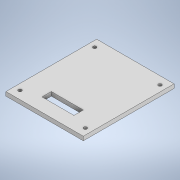
# Autodesk Inventor part: Podkladka
Saved by Autodesk Inventor 2021 (Build 250183000, 183)
## iProperties
Created: 2021-01-18
Part Number: Podkladka
Material: Generic
Document SubType Name: Modeling
Designer: emili
Density: 1 g/cm^3
Appearance: Default
Author: emili
Autodesk Inventor part; units mm, degrees
ref_plane "YZ Plane" through (0, 0, 0) normal (1, 0, 0) x (0, 1, 0)
ref_plane "XZ Plane" through (0, 0, 0) normal (0, 1, 0) x (-1, 0, 0)
ref_plane "XY Plane" through (0, 0, 0) normal (0, 0, 1) x (1, 0, 0)
sketch "Sketch2" plane through (0, 0, 0) normal (0, 1, 0) x (-1, 0, 0)
  line L0 (8, 0) -> (8, -5)
  line L1 (32, 0) -> (32, -5)
  line L2 (32, -5) -> (8, -5)
  line L3 (8, -5) -> (8, 0)
  line L4 (32, 0) -> (32, -5)
  line L5 (-9, 0) -> (-9, 9)
  line L6 (-9, 9) -> (0, 9)
  line L7 (49, -44) -> (49, -53)
  line L8 (49, -53) -> (40, -53)
  line L9 (-9, 9) -> (49, 9)
  line L10 (49, 9) -> (49, -53)
  line L11 (49, -53) -> (-9, -53)
  line L12 (-9, -53) -> (-9, 9)
  line L13 (8, 0) -> (8, 2)
  line L14 (8, 2) -> (32, 2)
  line L15 (32, 2) -> (32, 0)
  line L16 (32, 2) -> (8, 2)
  line L17 (8, 2) -> (8, -5)
  line L18 (8, -5) -> (32, -5)
  line L19 (32, -5) -> (32, 2)
  point P0 (0, 0)
  constraints: 40 end point, 6 parallel, 3 horizontal, 3 perpendicular
extrude "Extrusion1" add sketch "Sketch2" along normal blind 3
sketch "Sketch3" plane through (-49, 0, 9) normal (0, 0, 1) x (1, 0, 0)
  line L0 (0, 0) -> (0, 3) projected
  line L1 (58, 0) -> (58, 3) projected
  line L2 (0, 3) -> (58, 3)
  line L3 (58, 3) -> (58, 0)
  line L4 (58, 0) -> (0, 0)
  line L5 (0, 0) -> (0, 3)
  point P0 (49, 0)
  constraints: 8 end point, 2 parallel, 1 horizontal, 1 perpendicular
extrude "Extrusion2" add sketch "Sketch3" along normal blind 3
sketch "Sketch4" plane through (9, 0, -53) normal (0, 0, -1) x (-1, 0, 0)
  line L0 (58, 3) -> (58, 0) projected
  line L1 (58, 0) -> (0, 0) projected
  line L2 (58, 3) -> (0, 3)
  line L3 (0, 3) -> (0, 0)
  line L4 (0, 0) -> (58, 0)
  line L5 (58, 0) -> (58, 3)
  point P0 (9, 0)
  constraints: 8 end point, 2 parallel, 1 horizontal, 1 perpendicular
extrude "Extrusion3" add sketch "Sketch4" along normal blind 3
sketch "Sketch5" plane through (0, 3, 0) normal (0, 1, 0) x (1, 0, 0)
  line L0 (9, -12) -> (0, -12)
  line L1 (0, -12) -> (0, 0)
  line L2 (0, 0) -> (9, 0)
  line L3 (9, 0) -> (9, -12)
  line L4 (-49, -12) -> (-49, 56) projected
  line L5 (-49, 56) -> (-40, 56)
  line L6 (-40, 56) -> (-40, 44)
  line L7 (-40, 44) -> (-49, 44)
  line L8 (-49, 44) -> (-49, 56)
  line L9 (9, 56) -> (0, 56)
  line L10 (0, 56) -> (0, 44)
  line L11 (0, 44) -> (9, 44)
  line L12 (9, 44) -> (9, 56)
  circle A0 centre (-44.5, 50) radius 1.25
  circle A1 centre (4.5, 50) radius 1.25
  circle A2 centre (4.5, -6) radius 1.25
  line L13 (-49, -12) -> (-40, -12)
  line L14 (-40, -12) -> (-40, 0)
  line L15 (-40, 0) -> (-49, 0)
  line L16 (-49, 0) -> (-49, -12)
  circle A3 centre (-44.5, -6) radius 1.25
  dimension "d16" = 9
  dimension "d17" = 12
  dimension "d18" = 9
  dimension "d19" = 12
  dimension "d21" = 2.5
  dimension "d22" = 2.5
  dimension "d23" = 2.5
  dimension "d24" = 2.5
  constraints: 32 end point, 8 parallel, 4 centre point, 4 horizontal, 4 perpendicular, 4 point on line
  measures "d16" distance of L1.end L2.end
  measures "d17" distance of L0.end L1.end
  measures "d18" distance of L6.end L7.end
  measures "d19" distance of L5.end L6.end
  measures "d21" diameter of A0
  measures "d22" diameter of A1
  measures "d23" diameter of A2
  measures "d24" diameter of A3
extrude "Extrusion4" cut sketch "Sketch5" against normal blind 5 contours A0 | A1 | A2 | A3
body "Solid1"
